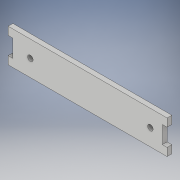
# Autodesk Inventor part: Tope riel motor 2
Saved by Autodesk Inventor 2019 (Build 230136000, 136)
## iProperties
Created: 2020-02-01
Part Number: Tope riel motor 2
Material: Generic
Document SubType Name: Modeling
Designer: Elías Sánchez
Density: 1 g/cm^3
Appearance: Default
Author: Elías Sánchez
Autodesk Inventor part; units mm, degrees
ref_plane "YZ Plane" through (0, 0, 0) normal (1, 0, 0) x (0, 1, 0)
ref_plane "XZ Plane" through (0, 0, 0) normal (0, 1, 0) x (-1, 0, 0)
ref_plane "XY Plane" through (0, 0, 0) normal (0, 0, 1) x (1, 0, 0)
sketch "Sketch1" plane through (0, 0, 0) normal (0, 0, 1) x (1, 0, 0)
  line L0 (-23, 42) -> (177, 42)
  line L1 (177, 0) -> (-23, 0)
  line L2 (-63, 0) -> (217, 0) projected
  line L3 (-23, 42) -> (-23, 32)
  line L4 (-23, 32) -> (-17, 32)
  line L5 (-17, 32) -> (-17, 10)
  line L6 (-17, 10) -> (-23, 10)
  line L7 (-23, 10) -> (-23, 0)
  line L8 (177, 42) -> (177, 32)
  line L9 (177, 32) -> (171, 32)
  line L10 (171, 32) -> (171, 10)
  line L11 (171, 10) -> (177, 10)
  line L12 (177, 10) -> (177, 0)
  circle A0 centre (156, 21) radius 3.5
  circle A1 centre (5, 21) radius 3.5
  point P0 (0, 0)
  point P1 (0, 0)
  dimension "d31" = 200
  dimension "d35" = 6
  dimension "d36" = 10
  dimension "d37" = 10
  dimension "d38" = 23
  dimension "d39" = 10
  dimension "d40" = 10
  dimension "d41" = 6
  dimension "d42" = 7
  dimension "d43" = 15
  dimension "d44" = 21
  dimension "d45" = 42
  dimension "d46" = 10
  dimension "d47" = 7
  dimension "d48" = 21
  dimension "d49" = 28
  constraints: 24 end point, 8 perpendicular, 2 centre point, 2 coincident, 2 point on line, 2 vertical, 1 horizontal, 1 parallel
  measures "d31" distance of L0.start L0.end
  measures "d35" distance of L5.end L6.end
  measures "d36" distance between parallel lines of L2 L6
  measures "d37" distance between parallel lines of L0 L4
  measures "d38" distance from line of point (0, 0) L7
  measures "d39" distance of L0.end L8.end
  measures "d40" distance of L11.end L1.start
  measures "d41" distance of L8.end L9.end
  measures "d42" diameter of A0
  measures "d43" distance from line of L10 A0.centre
  measures "d44" distance from line of A0.centre L2
  measures "d45" distance between parallel lines of L2 L0
  measures "d46" distance between parallel lines of L2 L11
  measures "d47" diameter of A1
  measures "d48" distance from line of L1 A1.centre
  measures "d49" distance from line of L3 A1.centre
extrude "Extrusion3" add sketch "Sketch1" along normal blind 6
equation "\"d37\" = d36"
equation "\"d39\" = d36"
equation "\"d40\" = d39"
equation "\"d41\" = d35"
equation "\"d47\" = d42"
equation "\"d48\" = d44"
body "Solid3"
